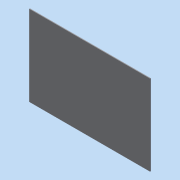
# Autodesk Inventor part: Fotofab_panel_16x12in
Saved by Autodesk Inventor 2014 (Build 180170000, 170)
## iProperties
Created: 2014-04-10
Part Number: Fotofab_panel_16x12in
Material: Generic
Document SubType Name: Sheet Metal
Designer: RDavis
Density: 1 g/cm^3
Sheet Metal Rule: Default
Appearance: Default
Author: RDavis
Autodesk Inventor part; units mm, degrees
ref_plane "YZ Plane" through (0, 0, 0) normal (1, 0, 0) x (0, 1, 0)
ref_plane "XZ Plane" through (0, 0, 0) normal (0, 1, 0) x (-1, 0, 0)
ref_plane "XY Plane" through (0, 0, 0) normal (0, 0, 1) x (1, 0, 0)
sketch "Sketch1" plane through (0, 0, 0) normal (0, 0, 1) x (1, 0, 0)
  line L0 (0, 118.1576) -> (0, 0)
  line L1 (0, 0) -> (122.0636, 0)
  line L2 (-228.6, 152.4) -> (228.6, 152.4)
  line L3 (228.6, 152.4) -> (228.6, -152.4)
  line L4 (228.6, -152.4) -> (-228.6, -152.4)
  line L5 (-228.6, -152.4) -> (-228.6, 152.4)
  dimension "d0" = 457.2
  dimension "d1" = 304.8
  measures "d0" distance of L2.start L2.end
  measures "d1" distance of L2.end L3.end
extrude "Plate1" add sketch "Sketch1" along normal blind 3.048
equation "\"BendRadius\" = Thickness"
equation "\"BendReliefWidth\" = Thickness"
equation "\"BendReliefDepth\" = 0.5 * Thickness"
equation "\"CornerReliefSize\" = 4 * Thickness"
equation "\"MinimumRemnant\" = 2 * Thickness"
equation "\"TransitionRadius\" = BendRadius"
equation "\"JacobiRadiusSize\" = BendRadius"
equation "\"GapSize\" = Thickness"
equation "\"d2\" = BendRadius"
equation "\"Thickness\" = 3.048"
body "Solid1"
